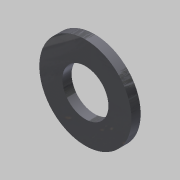
# Autodesk Inventor part: MSK01-08
Saved by Autodesk Inventor 2013 (Build 170138000, 138)
## iProperties
Created: 2012-01-24
Part Number: MSK01-08
Material: Steel, Mild
Document SubType Name: Modeling
Designer: ERF
Mass: 0.462992 g
Surface Area: 1.64934 cm^2
Volume: 0.0589049 cm^3
Density: 7.86 g/cm^3
Description: Shim 5mm 10mm 1mm Thk
Stock Number: B18026
Vendor: buildlog.net
Author: ERF
Title: Precision Washer (1mm thick)
Autodesk Inventor part; units mm, degrees
ref_plane "YZ Plane" through (0, 0, 0) normal (1, 0, 0) x (0, 1, 0)
ref_plane "XZ Plane" through (0, 0, 0) normal (0, 1, 0) x (-1, 0, 0)
ref_plane "XY Plane" through (0, 0, 0) normal (0, 0, 1) x (1, 0, 0)
sketch "Sketch1" plane through (0, 0, 0) normal (0, 0, 1) x (1, 0, 0)
  circle A0 centre (0, 0) radius 2.5
  circle A1 centre (0, 0) radius 5
  dimension "d0" = 5
  dimension "d1" = 10
  constraints: 2 centre point, 1 coincident
  measures "d0" diameter of A0
  measures "d1" diameter of A1
extrude "Extrusion1" add sketch "Sketch1" along normal blind 1
body "Solid1"
